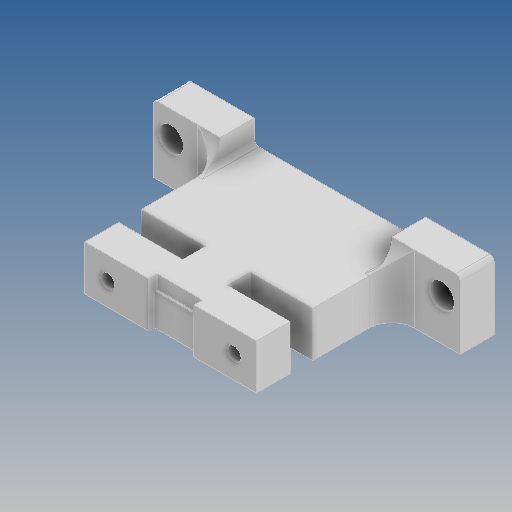
# Autodesk Inventor part: 0008-30-012
Saved by Autodesk Inventor 2020 (Build 240168000, 168)
## iProperties
Created: 2021-06-01
Part Number: 0008-30-012
Material: Generic
Document SubType Name: Modeling
Designer: Iulian Bors
Density: 1 g/cm^3
Appearance: Default
Author: Iulian Bors
Subject: 012
Autodesk Inventor part; units mm, degrees
note: some values were not read from the file. Chosen so that the rebuilt part matches the saved one: direction of "Hole2".
ref_plane "YZ Plane" through (0, 0, 0) normal (1, 0, 0) x (0, 1, 0)
ref_plane "XZ Plane" through (0, 0, 0) normal (0, 1, 0) x (-1, 0, 0)
ref_plane "XY Plane" through (0, 0, 0) normal (0, 0, 1) x (1, 0, 0)
sketch "Sketch1" plane through (0, 0, 0) normal (0, 0, 1) x (1, 0, 0)
  line L0 (-68, 15) -> (68, 15)
  line L1 (68, 15) -> (68, -15)
  line L2 (68, -15) -> (-68, -15)
  line L3 (-68, -15) -> (-68, 15)
  point P0 (0, 0)
  point P1 (-68, 0)
  point P2 (0, 15)
  dimension "d0" = 136
  dimension "d1" = 30
  constraints: 8 end point, 2 midpoint, 2 parallel, 1 horizontal, 1 horizontal alignment, 1 perpendicular, 1 vertical alignment
  measures "d0" distance of L0.start L0.end
  measures "d1" distance of L2.end L0.start
extrude "Extrusion1" add sketch "Sketch1" along normal blind 15
sketch "Sketch2" plane through (0, 0, 0) normal (0, 0, -1) x (-1, 0, 0)
  line L0 (-35.6981, 5) -> (36.3019, 5) projected
  line L1 (38.3019, 7) -> (38.3019, 13) projected
  line L2 (-37.6981, 13) -> (-37.6981, 7) projected
  line L3 (38.3019, 5) -> (-37.6981, 5)
  line L4 (-37.6981, 5) -> (-37.6981, 15)
  line L5 (-37.6981, 15) -> (38.3019, 15)
  line L6 (38.3019, 15) -> (38.3019, 5)
  line L7 (-68, 15) -> (68, 15) projected
  point P0 (0, 0)
  constraints: 8 end point, 4 collinear, 2 parallel, 1 horizontal, 1 perpendicular
extrude "Extrusion2" cut sketch "Sketch2" against normal through all
fillet "Fillet1" radius 2 2 edges at (68, 15, 7.5) (-68, 15, 7.5)
sketch "Sketch3" plane through (0, 0, 15) normal (0, 0, 1) x (1, 0, 0)
  line L0 (37.6981, -15) -> (-38.3019, -15)
  line L1 (-38.3019, -15) -> (-38.3019, 5)
  line L2 (-38.3019, 5) -> (37.6981, 5)
  line L3 (37.6981, 5) -> (37.6981, -15)
  line L4 (37.6981, 15) -> (37.6981, 5) projected
  line L5 (-38.3019, 5) -> (-38.3019, 15) projected
  line L6 (37.6981, 5) -> (-38.3019, 5) projected
  line L7 (-68, -15) -> (68, -15) projected
  point P0 (0, 0)
  constraints: 8 end point, 4 collinear, 2 parallel, 1 horizontal, 1 perpendicular
extrude "Extrusion3" add sketch "Sketch3" along normal blind 60
fillet "Fillet2" radius 10 2 edges at (-38.3019, -5, 15) (37.6981, -5, 15)
sketch "Sketch5" plane through (0, 0, 0) normal (1, 0, 0) x (0, 1, 0)
  line L0 (-7.23, 74.85) -> (-20.53, 74.85)
  line L1 (-0.53, 74.9229) -> (-7.23, 74.9229) projected
  line L2 (7, 71.6) -> (-0.53, 71.6)
  line L3 (-0.53, 72.825) -> (-5.23, 72.825) projected
  line L4 (-0.53, 71.6) -> (-0.53, 74.9229)
  line L5 (5, 75) -> (-15, 75) projected
  line L6 (5, 25) -> (5, 75) projected
  line L7 (5, 71.3) -> (-0.83, 71.3)
  line L8 (-0.83, 71.3) -> (-0.83, 74.6229)
  line L9 (-0.83, 74.6229) -> (-15.9201, 74.6229)
  line L10 (-15, 25) -> (-15, 75) projected
  line L11 (-15, 74.6229) -> (-15, 75)
  line L12 (-15, 75) -> (5, 75)
  line L13 (-0.83, 72.525) -> (-15, 72.525)
  line L14 (-15, 25) -> (-15, 75) projected
  point P0 (0, 0)
  dimension "d10" = 0.3
  dimension "d11" = 0.3
  dimension "d12" = 0.3
  dimension "d15" = 0.3
  constraints: 18 end point, 5 point on line, 3 parallel, 3 perpendicular, 2 horizontal, 1 collinear, 4 other
  measures "d10" distance between parallel lines of L7 L2
  measures "d11" distance from line of L3.start L8
  measures "d12" distance between parallel lines of L1 L9
  measures "d15" distance between parallel lines of L13 L3
extrude "Extrusion4" cut sketch "Sketch5" along normal mid plane 20
sketch "Sketch6" plane through (0, 0, 15) normal (0, 0, 1) x (1, 0, 0)
  circle A0 centre (-60.3019, 3.25) radius 8 projected
  circle A1 centre (59.6981, 3.25) radius 8 projected
  point P0 (0, 0)
hole "Hole1" at (-60.3019, 3.25, 15) at (59.6981, 3.25, 15) direction (0, 0, -1) diameter 11 end through all
sketch "Sketch7" plane through (-68, -15, 0) normal (0, -1, 0) x (1, 0, 0)
  line L0 (105.6981, 50) -> (78, 50)
  line L1 (78, 50) -> (78, 60)
  line L2 (78, 60) -> (105.6981, 60)
  line L3 (105.6981, 60) -> (105.6981, 50)
  line L4 (58, 50) -> (29.6981, 50)
  line L5 (29.6981, 50) -> (29.6981, 60)
  line L6 (29.6981, 60) -> (58, 60)
  line L7 (58, 60) -> (58, 50)
  line L8 (78, 75) -> (105.6981, 75) projected
  line L9 (29.6981, 25) -> (29.6981, 75) projected
  line L10 (58, 72.525) -> (58, 75) projected
  line L11 (78, 75) -> (78, 72.525) projected
  line L12 (105.6981, 25) -> (105.6981, 75) projected
  point P0 (68, 0)
  dimension "d23" = 10
  dimension "d24" = 15
  dimension "d25" = 27.6981
  dimension "d26" = 28.3019
  constraints: 16 end point, 5 collinear, 4 parallel, 2 horizontal, 2 perpendicular, 1 point on line
  measures "d23" distance of L2.end L0.start
  measures "d24" distance between parallel lines of L8 L2
  measures "d25" distance of L8.start L8.end
  measures "d26" distance of L5.end L6.end
extrude "Extrusion5" cut sketch "Sketch7" against normal blind 20
fillet "Fillet3" radius 2 2 edges at (-38.3019, 5, 7.5) (37.6981, 5, 7.5)
sketch "Sketch8" plane through (0, 0, 75) normal (0, 0, 1) x (1, 0, 0)
  line L0 (37.6981, -15) -> (37.6981, 5) projected
  line L1 (-38.3019, 5) -> (-38.3019, -15) projected
  point P0 (0, 0)
  point P1 (-28.3019, -5)
  point P2 (27.6981, -5)
  point P3 (37.6981, -5)
  point P4 (-38.3019, -5)
  dimension "d30" = 10
  dimension "d31" = 10
  constraints: 2 horizontal alignment, 2 midpoint
  measures "d30" distance from line of L1 point (-28.302, -5)
  measures "d31" distance from line of L0 point (27.698, -5)
hole "Hole2" at (-28.3019, -5, 75) at (27.6981, -5, 75) direction (0, 0, -1) diameter 6 depth 15
fillet "Fillet4" radius 10 2 edges at (-42.3019, 5, 15) (41.6981, 5, 15)
body "Solid1"
